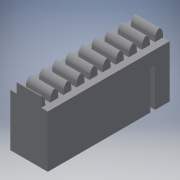
# Autodesk Inventor part: Alligator_Rack
Saved by Autodesk Inventor 2016 (Build 200138000, 138)
## iProperties
Created: 2017-05-22
Part Number: Alligator_Rack
Material: Generic
Document SubType Name: Modeling
Designer: nazardio000
Density: 1 g/cm^3
Appearance: Default
Author: nazardio000
Autodesk Inventor part; units mm, degrees
ref_plane "YZ Plane" through (0, 0, 0) normal (1, 0, 0) x (0, 1, 0)
ref_plane "XZ Plane" through (0, 0, 0) normal (0, 1, 0) x (-1, 0, 0)
ref_plane "XY Plane" through (0, 0, 0) normal (0, 0, 1) x (1, 0, 0)
sketch "Sketch2" plane through (0, 0, 0) normal (1, 0, 0) x (0, 1, 0)
  line L0 (-5.5245, 31.75) -> (-5.5245, -31.75)
  line L1 (-5.5245, -31.75) -> (5.5245, -31.75)
  line L2 (5.5245, -31.75) -> (5.5245, 31.75)
  line L3 (5.5245, 31.75) -> (-5.5245, 31.75)
  line L4 (-5.5245, 31.75) -> (5.5245, -31.75) construction
  line L5 (-5.5245, -31.75) -> (5.5245, 31.75) construction
  point P0 (0, 0)
  dimension "d4" = 63.5
  dimension "d5" = 11.049
  constraints: 12 end point, 2 midpoint, 2 parallel, 1 perpendicular, 1 vertical
  measures "d4" distance of L0.start L0.end
  measures "d5" distance of L1.end L0.end
extrude "Extrusion2" add sketch "Sketch2" along normal mid plane 9.779
sketch "Sketch3" plane through (0, 0, 0) normal (1, 0, 0) x (0, 1, 0)
  line L0 (5.5245, -31.75) -> (5.5245, 31.75) projected
  line L1 (5.5245, 31.9532) -> (5.5245, 29.4132)
  line L2 (5.5245, 31.9532) -> (5.5245, 29.4132)
  arc A0 (8.0645, 30.8543) -> (6.7945, 31.629) centre (6.3804, 29.5218) ccw
  line L3 (8.0645, 30.6737) -> (7.6408, 30.6737)
  arc A1 (6.7945, 29.7184) -> (8.0645, 30.4931) centre (6.3804, 31.8256) ccw
  line L4 (8.0645, 30.8543) -> (8.0645, 30.4931)
  line L5 (5.5245, 31.75) -> (5.5245, -31.75)
  arc A2 (8.0642, -1.6042) -> (8.0645, -1.6033) centre (6.6313, -1.0154) ccw
  line L6 (6.7945, 31.629) -> (5.5245, 31.7489)
  line L7 (6.7945, 29.7184) -> (5.5245, 29.5986)
  line L8 (5.5245, 31.7489) -> (6.7945, 31.629)
  line L9 (6.7945, 29.7184) -> (5.5245, 29.5986)
  line L10 (5.5245, 29.5986) -> (5.5245, 31.7489)
  arc A3 (8.0645, 30.8543) -> (6.7945, 31.629) centre (6.3804, 29.5218) ccw
  arc A4 (6.7945, 29.7184) -> (8.0645, 30.4931) centre (6.3804, 31.8256) ccw
  line L11 (8.0645, 30.8543) -> (8.0645, 30.4931)
  line L12 (8.0645, 27.2655) -> (7.6408, 27.2655)
  line L13 (8.0645, 27.4461) -> (8.0645, 27.0848)
  line L14 (8.0645, 27.4461) -> (8.0645, 27.0848)
  arc A5 (6.7945, 26.3101) -> (8.0645, 27.0848) centre (6.3804, 28.4173) ccw
  arc A6 (8.0645, 27.4461) -> (6.7945, 28.2208) centre (6.3804, 26.1136) ccw
  arc A7 (6.7945, 26.3101) -> (8.0645, 27.0848) centre (6.3804, 28.4173) ccw
  arc A8 (8.0645, 27.4461) -> (6.7945, 28.2208) centre (6.3804, 26.1136) ccw
  line L15 (5.5245, 28.3417) -> (5.5245, -35.1582)
  line L16 (5.5245, 28.5449) -> (5.5245, 26.0049)
  line L17 (6.7945, 26.3101) -> (5.5245, 26.1903)
  line L18 (5.5245, 28.3406) -> (6.7945, 28.2208)
  line L19 (6.7945, 26.3101) -> (5.5245, 26.1903)
  line L20 (5.5245, 26.1903) -> (5.5245, 28.3406)
  line L21 (5.5245, 28.5449) -> (5.5245, 26.0049)
  line L22 (6.7945, 28.2208) -> (5.5245, 28.3406)
  line L23 (8.0645, 23.8572) -> (7.6408, 23.8572)
  line L24 (8.0645, 24.0378) -> (8.0645, 23.6766)
  line L25 (8.0645, 24.0378) -> (8.0645, 23.6766)
  arc A9 (6.7945, 22.9019) -> (8.0645, 23.6766) centre (6.3804, 25.0091) ccw
  arc A10 (8.0645, 24.0378) -> (6.7945, 24.8125) centre (6.3804, 22.7053) ccw
  arc A11 (6.7945, 22.9019) -> (8.0645, 23.6766) centre (6.3804, 25.0091) ccw
  arc A12 (8.0645, 24.0378) -> (6.7945, 24.8125) centre (6.3804, 22.7053) ccw
  line L26 (5.5245, 24.9335) -> (5.5245, -38.5665)
  line L27 (5.5245, 25.1367) -> (5.5245, 22.5967)
  line L28 (6.7945, 22.9019) -> (5.5245, 22.782)
  line L29 (5.5245, 24.9324) -> (6.7945, 24.8125)
  line L30 (6.7945, 22.9019) -> (5.5245, 22.782)
  line L31 (5.5245, 22.782) -> (5.5245, 24.9324)
  line L32 (5.5245, 25.1367) -> (5.5245, 22.5967)
  line L33 (6.7945, 24.8125) -> (5.5245, 24.9324)
  line L34 (8.0645, 20.449) -> (7.6408, 20.449)
  line L35 (8.0645, 20.6296) -> (8.0645, 20.2683)
  line L36 (8.0645, 20.6296) -> (8.0645, 20.2683)
  arc A13 (6.7945, 19.4936) -> (8.0645, 20.2683) centre (6.3804, 21.6008) ccw
  arc A14 (8.0645, 20.6296) -> (6.7945, 21.4043) centre (6.3804, 19.2971) ccw
  arc A15 (6.7945, 19.4936) -> (8.0645, 20.2683) centre (6.3804, 21.6008) ccw
  arc A16 (8.0645, 20.6296) -> (6.7945, 21.4043) centre (6.3804, 19.2971) ccw
  line L37 (5.5245, 21.5252) -> (5.5245, -41.9747)
  line L38 (5.5245, 21.7284) -> (5.5245, 19.1884)
  line L39 (6.7945, 19.4936) -> (5.5245, 19.3738)
  line L40 (5.5245, 21.5241) -> (6.7945, 21.4043)
  line L41 (6.7945, 19.4936) -> (5.5245, 19.3738)
  line L42 (5.5245, 19.3738) -> (5.5245, 21.5241)
  line L43 (5.5245, 21.7284) -> (5.5245, 19.1884)
  line L44 (6.7945, 21.4043) -> (5.5245, 21.5241)
  line L45 (8.0645, 17.0407) -> (7.6408, 17.0407)
  line L46 (8.0645, 17.2213) -> (8.0645, 16.8601)
  line L47 (8.0645, 17.2213) -> (8.0645, 16.8601)
  arc A17 (6.7945, 16.0854) -> (8.0645, 16.8601) centre (6.3804, 18.1926) ccw
  arc A18 (8.0645, 17.2213) -> (6.7945, 17.996) centre (6.3804, 15.8888) ccw
  arc A19 (6.7945, 16.0854) -> (8.0645, 16.8601) centre (6.3804, 18.1926) ccw
  arc A20 (8.0645, 17.2213) -> (6.7945, 17.996) centre (6.3804, 15.8888) ccw
  line L48 (5.5245, 18.117) -> (5.5245, -45.383)
  line L49 (5.5245, 18.3202) -> (5.5245, 15.7802)
  line L50 (6.7945, 16.0854) -> (5.5245, 15.9655)
  line L51 (5.5245, 18.1159) -> (6.7945, 17.996)
  line L52 (6.7945, 16.0854) -> (5.5245, 15.9655)
  line L53 (5.5245, 15.9655) -> (5.5245, 18.1159)
  line L54 (5.5245, 18.3202) -> (5.5245, 15.7802)
  line L55 (6.7945, 17.996) -> (5.5245, 18.1159)
  line L56 (8.0645, 13.6324) -> (7.6408, 13.6324)
  line L57 (8.0645, 13.8131) -> (8.0645, 13.4518)
  line L58 (8.0645, 13.8131) -> (8.0645, 13.4518)
  arc A21 (6.7945, 12.6771) -> (8.0645, 13.4518) centre (6.3804, 14.7843) ccw
  arc A22 (8.0645, 13.8131) -> (6.7945, 14.5878) centre (6.3804, 12.4806) ccw
  arc A23 (6.7945, 12.6771) -> (8.0645, 13.4518) centre (6.3804, 14.7843) ccw
  arc A24 (8.0645, 13.8131) -> (6.7945, 14.5878) centre (6.3804, 12.4806) ccw
  line L59 (5.5245, 14.7087) -> (5.5245, -48.7912)
  line L60 (5.5245, 14.9119) -> (5.5245, 12.3719)
  line L61 (6.7945, 12.6771) -> (5.5245, 12.5573)
  line L62 (5.5245, 14.7076) -> (6.7945, 14.5878)
  line L63 (6.7945, 12.6771) -> (5.5245, 12.5573)
  line L64 (5.5245, 12.5573) -> (5.5245, 14.7076)
  line L65 (5.5245, 14.9119) -> (5.5245, 12.3719)
  line L66 (6.7945, 14.5878) -> (5.5245, 14.7076)
  line L67 (8.0645, 10.2242) -> (7.6408, 10.2242)
  line L68 (8.0645, 10.4048) -> (8.0645, 10.0436)
  line L69 (8.0645, 10.4048) -> (8.0645, 10.0436)
  arc A25 (6.7945, 9.2689) -> (8.0645, 10.0436) centre (6.3804, 11.3761) ccw
  arc A26 (8.0645, 10.4048) -> (6.7945, 11.1795) centre (6.3804, 9.0723) ccw
  arc A27 (6.7945, 9.2689) -> (8.0645, 10.0436) centre (6.3804, 11.3761) ccw
  arc A28 (8.0645, 10.4048) -> (6.7945, 11.1795) centre (6.3804, 9.0723) ccw
  line L70 (5.5245, 11.3005) -> (5.5245, -52.1995)
  line L71 (5.5245, 11.5037) -> (5.5245, 8.9637)
  line L72 (6.7945, 9.2689) -> (5.5245, 9.149)
  line L73 (5.5245, 11.2994) -> (6.7945, 11.1795)
  line L74 (6.7945, 9.2689) -> (5.5245, 9.149)
  line L75 (5.5245, 9.149) -> (5.5245, 11.2994)
  line L76 (5.5245, 11.5037) -> (5.5245, 8.9637)
  line L77 (6.7945, 11.1795) -> (5.5245, 11.2994)
  line L78 (8.0645, 6.8159) -> (7.6408, 6.8159)
  line L79 (8.0645, 6.9966) -> (8.0645, 6.6353)
  line L80 (8.0645, 6.9966) -> (8.0645, 6.6353)
  arc A29 (6.7945, 5.8606) -> (8.0645, 6.6353) centre (6.3804, 7.9678) ccw
  arc A30 (8.0645, 6.9966) -> (6.7945, 7.7713) centre (6.3804, 5.6641) ccw
  arc A31 (6.7945, 5.8606) -> (8.0645, 6.6353) centre (6.3804, 7.9678) ccw
  arc A32 (8.0645, 6.9966) -> (6.7945, 7.7713) centre (6.3804, 5.6641) ccw
  line L81 (5.5245, 7.8922) -> (5.5245, -55.6077)
  line L82 (5.5245, 8.0954) -> (5.5245, 5.5554)
  line L83 (6.7945, 5.8606) -> (5.5245, 5.7408)
  line L84 (5.5245, 7.8911) -> (6.7945, 7.7713)
  line L85 (6.7945, 5.8606) -> (5.5245, 5.7408)
  line L86 (5.5245, 5.7408) -> (5.5245, 7.8911)
  line L87 (5.5245, 8.0954) -> (5.5245, 5.5554)
  line L88 (6.7945, 7.7713) -> (5.5245, 7.8911)
  line L89 (8.0645, 3.4077) -> (7.6408, 3.4077)
  line L90 (8.0645, 3.5883) -> (8.0645, 3.2271)
  line L91 (8.0645, 3.5883) -> (8.0645, 3.2271)
  arc A33 (6.7945, 2.4524) -> (8.0645, 3.2271) centre (6.3804, 4.5596) ccw
  arc A34 (8.0645, 3.5883) -> (6.7945, 4.363) centre (6.3804, 2.2558) ccw
  arc A35 (6.7945, 2.4524) -> (8.0645, 3.2271) centre (6.3804, 4.5596) ccw
  arc A36 (8.0645, 3.5883) -> (6.7945, 4.363) centre (6.3804, 2.2558) ccw
  line L92 (5.5245, 4.484) -> (5.5245, -59.016)
  line L93 (5.5245, 4.6872) -> (5.5245, 2.1472)
  line L94 (6.7945, 2.4524) -> (5.5245, 2.3325)
  line L95 (5.5245, 4.4829) -> (6.7945, 4.363)
  line L96 (6.7945, 2.4524) -> (5.5245, 2.3325)
  line L97 (5.5245, 2.3325) -> (5.5245, 4.4829)
  line L98 (5.5245, 4.6872) -> (5.5245, 2.1472)
  line L99 (6.7945, 4.363) -> (5.5245, 4.4829)
  line L100 (8.0645, -0.0006) -> (7.6408, -0.0006)
  line L101 (8.0645, 0.1801) -> (8.0645, -0.1812)
  line L102 (8.0645, 0.1801) -> (8.0645, -0.1812)
  arc A37 (6.7945, -0.9559) -> (8.0645, -0.1812) centre (6.3804, 1.1513) ccw
  arc A38 (8.0645, 0.1801) -> (6.7945, 0.9548) centre (6.3804, -1.1524) ccw
  arc A39 (6.7945, -0.9559) -> (8.0645, -0.1812) centre (6.3804, 1.1513) ccw
  arc A40 (8.0645, 0.1801) -> (6.7945, 0.9548) centre (6.3804, -1.1524) ccw
  line L103 (5.5245, 1.0757) -> (5.5245, -62.4242)
  line L104 (5.5245, 1.2789) -> (5.5245, -1.2611)
  line L105 (6.7945, -0.9559) -> (5.5245, -1.0757)
  line L106 (5.5245, 1.0746) -> (6.7945, 0.9548)
  line L107 (6.7945, -0.9559) -> (5.5245, -1.0757)
  line L108 (5.5245, -1.0757) -> (5.5245, 1.0746)
  line L109 (5.5245, 1.2789) -> (5.5245, -1.2611)
  line L110 (6.7945, 0.9548) -> (5.5245, 1.0746)
  line L111 (8.0645, -3.4088) -> (7.6408, -3.4088)
  line L112 (8.0645, -3.2282) -> (8.0645, -3.5894)
  line L113 (8.0645, -3.2282) -> (8.0645, -3.5894)
  arc A41 (6.7945, -4.3641) -> (8.0645, -3.5894) centre (6.3804, -2.2569) ccw
  arc A42 (8.0645, -3.2282) -> (6.7945, -2.4535) centre (6.3804, -4.5607) ccw
  arc A43 (6.7945, -4.3641) -> (8.0645, -3.5894) centre (6.3804, -2.2569) ccw
  arc A44 (8.0645, -3.2282) -> (6.7945, -2.4535) centre (6.3804, -4.5607) ccw
  line L114 (5.5245, -2.3325) -> (5.5245, -65.8325)
  line L115 (5.5245, -2.1293) -> (5.5245, -4.6693)
  line L116 (6.7945, -4.3641) -> (5.5245, -4.484)
  line L117 (5.5245, -2.3337) -> (6.7945, -2.4535)
  line L118 (6.7945, -4.3641) -> (5.5245, -4.484)
  line L119 (5.5245, -4.484) -> (5.5245, -2.3337)
  line L120 (5.5245, -2.1293) -> (5.5245, -4.6693)
  line L121 (6.7945, -2.4535) -> (5.5245, -2.3337)
  line L122 (8.0645, -6.8171) -> (7.6408, -6.8171)
  line L123 (8.0645, -6.6364) -> (8.0645, -6.9977)
  line L124 (8.0645, -6.6364) -> (8.0645, -6.9977)
  arc A45 (6.7945, -7.7724) -> (8.0645, -6.9977) centre (6.3804, -5.6652) ccw
  arc A46 (8.0645, -6.6364) -> (6.7945, -5.8617) centre (6.3804, -7.9689) ccw
  arc A47 (6.7945, -7.7724) -> (8.0645, -6.9977) centre (6.3804, -5.6652) ccw
  arc A48 (8.0645, -6.6364) -> (6.7945, -5.8617) centre (6.3804, -7.9689) ccw
  line L125 (5.5245, -5.7408) -> (5.5245, -69.2407)
  line L126 (5.5245, -5.5376) -> (5.5245, -8.0776)
  line L127 (6.7945, -7.7724) -> (5.5245, -7.8922)
  line L128 (5.5245, -5.7419) -> (6.7945, -5.8617)
  line L129 (6.7945, -7.7724) -> (5.5245, -7.8922)
  line L130 (5.5245, -7.8922) -> (5.5245, -5.7419)
  line L131 (5.5245, -5.5376) -> (5.5245, -8.0776)
  line L132 (6.7945, -5.8617) -> (5.5245, -5.7419)
  line L133 (8.0645, -10.2253) -> (7.6408, -10.2253)
  line L134 (8.0645, -10.0447) -> (8.0645, -10.4059)
  line L135 (8.0645, -10.0447) -> (8.0645, -10.4059)
  arc A49 (6.7945, -11.1806) -> (8.0645, -10.4059) centre (6.3804, -9.0734) ccw
  arc A50 (8.0645, -10.0447) -> (6.7945, -9.27) centre (6.3804, -11.3772) ccw
  arc A51 (6.7945, -11.1806) -> (8.0645, -10.4059) centre (6.3804, -9.0734) ccw
  arc A52 (8.0645, -10.0447) -> (6.7945, -9.27) centre (6.3804, -11.3772) ccw
  line L136 (5.5245, -9.149) -> (5.5245, -72.649)
  line L137 (5.5245, -8.9458) -> (5.5245, -11.4858)
  line L138 (6.7945, -11.1806) -> (5.5245, -11.3005)
  line L139 (5.5245, -9.1502) -> (6.7945, -9.27)
  line L140 (6.7945, -11.1806) -> (5.5245, -11.3005)
  line L141 (5.5245, -11.3005) -> (5.5245, -9.1502)
  line L142 (5.5245, -8.9458) -> (5.5245, -11.4858)
  line L143 (6.7945, -9.27) -> (5.5245, -9.1502)
  line L144 (8.0645, -13.6336) -> (7.6408, -13.6336)
  line L145 (8.0645, -13.4529) -> (8.0645, -13.8142)
  line L146 (8.0645, -13.4529) -> (8.0645, -13.8142)
  arc A53 (6.7945, -14.5889) -> (8.0645, -13.8142) centre (6.3804, -12.4817) ccw
  arc A54 (8.0645, -13.4529) -> (6.7945, -12.6782) centre (6.3804, -14.7854) ccw
  arc A55 (6.7945, -14.5889) -> (8.0645, -13.8142) centre (6.3804, -12.4817) ccw
  arc A56 (8.0645, -13.4529) -> (6.7945, -12.6782) centre (6.3804, -14.7854) ccw
  line L147 (5.5245, -12.5573) -> (5.5245, -76.0572)
  line L148 (5.5245, -12.3541) -> (5.5245, -14.8941)
  line L149 (6.7945, -14.5889) -> (5.5245, -14.7087)
  line L150 (5.5245, -12.5584) -> (6.7945, -12.6782)
  line L151 (6.7945, -14.5889) -> (5.5245, -14.7087)
  line L152 (5.5245, -14.7087) -> (5.5245, -12.5584)
  line L153 (5.5245, -12.3541) -> (5.5245, -14.8941)
  line L154 (6.7945, -12.6782) -> (5.5245, -12.5584)
  line L155 (8.0645, -17.0418) -> (7.6408, -17.0418)
  line L156 (8.0645, -16.8612) -> (8.0645, -17.2224)
  line L157 (8.0645, -16.8612) -> (8.0645, -17.2224)
  arc A57 (6.7945, -17.9971) -> (8.0645, -17.2224) centre (6.3804, -15.8899) ccw
  arc A58 (8.0645, -16.8612) -> (6.7945, -16.0865) centre (6.3804, -18.1937) ccw
  arc A59 (6.7945, -17.9971) -> (8.0645, -17.2224) centre (6.3804, -15.8899) ccw
  arc A60 (8.0645, -16.8612) -> (6.7945, -16.0865) centre (6.3804, -18.1937) ccw
  line L158 (5.5245, -15.9655) -> (5.5245, -79.4655)
  line L159 (5.5245, -15.7623) -> (5.5245, -18.3023)
  line L160 (6.7945, -17.9971) -> (5.5245, -18.117)
  line L161 (5.5245, -15.9667) -> (6.7945, -16.0865)
  line L162 (6.7945, -17.9971) -> (5.5245, -18.117)
  line L163 (5.5245, -18.117) -> (5.5245, -15.9667)
  line L164 (5.5245, -15.7623) -> (5.5245, -18.3023)
  line L165 (6.7945, -16.0865) -> (5.5245, -15.9667)
  line L166 (8.0645, -20.4501) -> (7.6408, -20.4501)
  line L167 (8.0645, -20.2694) -> (8.0645, -20.6307)
  line L168 (8.0645, -20.2694) -> (8.0645, -20.6307)
  arc A61 (6.7945, -21.4054) -> (8.0645, -20.6307) centre (6.3804, -19.2982) ccw
  arc A62 (8.0645, -20.2694) -> (6.7945, -19.4947) centre (6.3804, -21.6019) ccw
  arc A63 (6.7945, -21.4054) -> (8.0645, -20.6307) centre (6.3804, -19.2982) ccw
  arc A64 (8.0645, -20.2694) -> (6.7945, -19.4947) centre (6.3804, -21.6019) ccw
  line L169 (5.5245, -19.3738) -> (5.5245, -82.8737)
  line L170 (5.5245, -19.1706) -> (5.5245, -21.7106)
  line L171 (6.7945, -21.4054) -> (5.5245, -21.5252)
  line L172 (5.5245, -19.3749) -> (6.7945, -19.4947)
  line L173 (6.7945, -21.4054) -> (5.5245, -21.5252)
  line L174 (5.5245, -21.5252) -> (5.5245, -19.3749)
  line L175 (5.5245, -19.1706) -> (5.5245, -21.7106)
  line L176 (6.7945, -19.4947) -> (5.5245, -19.3749)
  line L177 (8.0645, -23.8583) -> (7.6408, -23.8583)
  line L178 (8.0645, -23.6777) -> (8.0645, -24.0389)
  line L179 (8.0645, -23.6777) -> (8.0645, -24.0389)
  arc A65 (6.7945, -24.8136) -> (8.0645, -24.0389) centre (6.3804, -22.7064) ccw
  arc A66 (8.0645, -23.6777) -> (6.7945, -22.903) centre (6.3804, -25.0102) ccw
  arc A67 (6.7945, -24.8136) -> (8.0645, -24.0389) centre (6.3804, -22.7064) ccw
  arc A68 (8.0645, -23.6777) -> (6.7945, -22.903) centre (6.3804, -25.0102) ccw
  line L180 (5.5245, -22.782) -> (5.5245, -86.282)
  line L181 (5.5245, -22.5788) -> (5.5245, -25.1188)
  line L182 (6.7945, -24.8136) -> (5.5245, -24.9335)
  line L183 (5.5245, -22.7832) -> (6.7945, -22.903)
  line L184 (6.7945, -24.8136) -> (5.5245, -24.9335)
  line L185 (5.5245, -24.9335) -> (5.5245, -22.7832)
  line L186 (5.5245, -22.5788) -> (5.5245, -25.1188)
  line L187 (6.7945, -22.903) -> (5.5245, -22.7832)
  line L188 (8.0645, -27.2666) -> (7.6408, -27.2666)
  line L189 (8.0645, -27.0859) -> (8.0645, -27.4472)
  line L190 (8.0645, -27.0859) -> (8.0645, -27.4472)
  arc A69 (6.7945, -28.2219) -> (8.0645, -27.4472) centre (6.3804, -26.1147) ccw
  arc A70 (8.0645, -27.0859) -> (6.7945, -26.3112) centre (6.3804, -28.4184) ccw
  arc A71 (6.7945, -28.2219) -> (8.0645, -27.4472) centre (6.3804, -26.1147) ccw
  arc A72 (8.0645, -27.0859) -> (6.7945, -26.3112) centre (6.3804, -28.4184) ccw
  line L191 (5.5245, -26.1903) -> (5.5245, -89.6902)
  line L192 (5.5245, -25.9871) -> (5.5245, -28.5271)
  line L193 (6.7945, -28.2219) -> (5.5245, -28.3417)
  line L194 (5.5245, -26.1914) -> (6.7945, -26.3112)
  line L195 (6.7945, -28.2219) -> (5.5245, -28.3417)
  line L196 (5.5245, -28.3417) -> (5.5245, -26.1914)
  line L197 (5.5245, -25.9871) -> (5.5245, -28.5271)
  line L198 (6.7945, -26.3112) -> (5.5245, -26.1914)
  line L199 (8.0645, -30.6748) -> (7.6408, -30.6748)
  line L200 (8.0645, -30.4942) -> (8.0645, -30.8554)
  line L201 (8.0645, -30.4942) -> (8.0645, -30.8554)
  arc A73 (6.7945, -31.6301) -> (8.0645, -30.8554) centre (6.3804, -29.5229) ccw
  arc A74 (8.0645, -30.4942) -> (6.7945, -29.7195) centre (6.3804, -31.8267) ccw
  arc A75 (6.7945, -31.6301) -> (8.0645, -30.8554) centre (6.3804, -29.5229) ccw
  arc A76 (8.0645, -30.4942) -> (6.7945, -29.7195) centre (6.3804, -31.8267) ccw
  line L202 (5.5245, -29.5985) -> (5.5245, -93.0985)
  line L203 (5.5245, -29.3953) -> (5.5245, -31.9353)
  line L204 (6.7945, -31.6301) -> (5.5245, -31.75)
  line L205 (5.5245, -29.5997) -> (6.7945, -29.7195)
  line L206 (6.7945, -31.6301) -> (5.5245, -31.75)
  line L207 (5.5245, -31.75) -> (5.5245, -29.5997)
  line L208 (5.5245, -29.3953) -> (5.5245, -31.9353)
  line L209 (6.7945, -29.7195) -> (5.5245, -29.5997)
  point P0 (0, 0)
  point P1 (6.7953, 29.7185)
  point P2 (6.7953, 26.3103)
  point P3 (6.7953, 22.902)
  point P4 (6.7953, 19.4938)
  point P5 (6.7953, 16.0855)
  point P6 (6.7953, 12.6773)
  point P7 (6.7953, 9.269)
  point P8 (6.7953, 5.8608)
  point P9 (6.7953, 2.4525)
  point P10 (6.7953, -0.9557)
  point P11 (6.7953, -4.364)
  point P12 (6.7953, -7.7722)
  point P13 (6.7953, -11.1805)
  point P14 (6.7953, -14.5887)
  point P15 (6.7953, -17.997)
  point P16 (6.7953, -21.4052)
  point P17 (6.7953, -24.8135)
  point P18 (6.7953, -28.2217)
  point P19 (6.7953, -31.63)
  dimension "d9" = 2.3368
  dimension "d63" = 84.61
  dimension "d64" = 84.61
  dimension "d74" = 3.4082
  constraints: 382 end point, 173 point on circle, 77 centre point, 19 coincident, 5 collinear, 3 symmetric about line, 2 concentric, 2 vertical, 1 horizontal, 595 other
  measures "d9" distance of L0.end L1.end
  measures "d63" angle of L0 L6
  measures "d64" angle of L0 L7
  measures "d74" distance of L1.end L16.end
sketch "Sketch4" plane through (-4.8895, -5.5245, -31.75) normal (0, -1, 0) x (1, 0, 0)
  line L0 (2.032, 0.0016) -> (7.747, 0.0016) projected
  line L1 (4.8895, 0.0016) -> (6.7945, 0.0016)
  line L2 (4.8895, 0.0016) -> (2.9845, 0.0016)
  line L3 (6.7945, 0.0016) -> (2.032, 0.0016)
  line L4 (2.9845, -0.9507) -> (6.7945, -0.9507)
  line L5 (6.7945, -0.9507) -> (6.7945, 0.0016)
  line L6 (6.7945, 0.0016) -> (6.7945, 2.5416)
  line L7 (7.747, 2.5416) -> (2.032, 2.5416) projected
  line L8 (2.032, 2.5416) -> (0, 2.5416)
  line L9 (0, 63.5) -> (0, 0) projected
  line L10 (6.7945, 2.5416) -> (9.779, 2.5416)
  line L11 (9.779, 0) -> (9.779, 63.5) projected
  line L12 (9.779, 2.5416) -> (9.779, 3.8116)
  line L13 (9.779, 3.8116) -> (0, 3.8116)
  line L14 (0, 2.5416) -> (0, 3.8116)
  line L15 (2.9845, 0.0016) -> (2.9845, -0.9507)
  line L16 (2.9845, 0.0016) -> (2.9845, 2.5416)
  line L17 (2.032, 2.5416) -> (2.9845, 2.5416)
  point P0 (4.8895, 31.75)
  dimension "d28" = 1.905
  dimension "d29" = 1.905
  dimension "d31" = 2.54
  dimension "d32" = 1.27
  constraints: 28 end point, 9 point on line, 2 collinear, 2 perpendicular, 1 horizontal, 1 midpoint, 1 parallel, 1 vertical
  measures "d28" distance of L1.start L1.end
  measures "d29" distance of L1.start L2.end
  measures "d31" distance of L1.end L6.end
  measures "d32" distance of L10.end L12.end
extrude "Extrusion4" cut sketch "Sketch4" against normal blind 10.16
sketch "Sketch5" plane through (-4.8895, -5.5245, 31.75) normal (0, -1, 0) x (1, 0, 0)
  line L0 (0, -59.6884) -> (9.779, -59.6884) projected
  line L1 (9.779, 0) -> (9.779, -59.6884) projected
  line L2 (9.779, 0) -> (0, 0) projected
  line L3 (0, -59.6884) -> (0, 0) projected
  line L4 (2.9845, -60.9584) -> (0, -60.9584) projected
  line L5 (0, -63.5) -> (0, -60.9584) projected
  line L6 (0, -63.5) -> (2.9845, -63.5) projected
  line L7 (2.9845, -63.5) -> (2.9845, -60.9584) projected
  line L8 (9.779, -60.9584) -> (6.7945, -60.9584) projected
  line L9 (6.7945, -60.9584) -> (6.7945, -63.5) projected
  line L10 (6.7945, -63.5) -> (9.779, -63.5) projected
  line L11 (9.779, -60.9584) -> (9.779, -63.5) projected
  point P0 (4.8895, -31.75)
extrude "Extrusion6" add sketch "Sketch5" along normal blind 2.54
sketch "Sketch6" plane through (4.8895, 0, 0) normal (1, 0, 0) x (0, 0, -1)
  line L0 (31.75, 5.5245) -> (31.75, -8.0645) projected
  line L1 (27.9384, 4.6355) -> (31.75, 4.6355)
  line L2 (31.75, 4.6355) -> (31.75, 2.0955)
  line L3 (31.75, 2.0955) -> (27.9384, 2.0955)
  line L4 (27.9384, 2.0955) -> (27.9384, 4.6355)
  point P0 (0, 0)
  dimension "d60" = 2.54
  constraints: 8 end point, 2 parallel, 1 horizontal, 1 perpendicular, 1 point on line
  measures "d60" distance of L3.end L1.start
extrude "Extrusion7" add sketch "Sketch6" against normal blind 9.779
extrude "Extrusion8" add sketch "Sketch3" along normal mid plane 6.35 contours L0 L6 A0 L4 A1 L7 | L0 L18 A6 L13 A5 L17 | L0 L29 A10 L24 A9 L28 | L0 L40 A14 L35 A13 L39 | L0 L51 A18 L46 A17 L50 | L0 L62 A22 L57 A21 L61 | L0 L73 A26 L68 A25 L72 | L0 L84 A30 L79 A29 L83 | L0 L95 A34 L90 A33 L94 | L0 L117 A2 A42 L112 A41 L116 | L0 L128 A46 L123 A45 L127 | L0 L139 A50 L134 A49 L138 | L0 L150 A54 L145 A53 L149 | L0 L161 A58 L156 A57 L160 | L0 L172 A62 L167 A61 L171 | L0 L183 A66 L178 A65 L182 | L0 L194 A70 L189 A69 L193 | L0 L205 A74 L200 A73 L204 | L117 A42 A2 | A2 A37 L105 L0 | L0 L106 A38 L101 L100 A2 | L100 L101 A37 A2
sketch "Sketch7" plane through (4.8895, 0, 0) normal (1, 0, 0) x (0, 0, -1)
  line L0 (29.2084, 2.0955) -> (31.75, 2.0955) projected
  line L1 (27.9384, 2.0955) -> (27.9384, -8.0645) projected
  line L2 (29.2084, 2.0955) -> (27.9384, 2.0955)
  line L3 (27.9384, 2.0955) -> (27.9384, -8.0645)
  line L4 (27.9384, -8.0645) -> (29.2084, -8.0645)
  line L5 (29.2084, -8.0645) -> (29.2084, 2.0955)
  line L6 (27.9384, -8.0645) -> (26.6684, -8.0645)
  line L7 (26.6684, -8.0645) -> (26.6684, 2.0955)
  line L8 (26.6684, 2.0955) -> (27.9384, 2.0955)
  line L9 (27.9384, 2.0955) -> (27.9384, -8.0645)
  point P0 (0, 0)
  dimension "d81" = 1.27
  constraints: 16 end point, 4 parallel, 2 horizontal, 2 perpendicular
  measures "d81" distance of L7.end L8.end
extrude "Extrusion9" add sketch "Sketch7" against normal blind 9.779 contours L2 L5 L4 L1
sketch "Sketch8" plane through (4.8895, 0, 0) normal (1, 0, 0) x (0, 0, -1)
  line L0 (31.75, -8.0645) -> (29.2084, -8.0645) projected
  line L1 (31.75, -8.0645) -> (27.94, -8.0645)
  line L2 (-31.75, -8.0645) -> (31.75, -8.0645) projected
  line L3 (27.94, -8.0645) -> (26.67, -8.0645)
  line L4 (27.94, -8.0645) -> (27.94, 2.0955)
  line L5 (27.94, 2.0955) -> (26.67, 2.0955)
  line L6 (26.67, 2.0955) -> (26.67, -8.0645)
  point P0 (0, 0)
  dimension "d84" = 3.81
  dimension "d85" = 1.27
  dimension "d86" = 10.16
  constraints: 10 end point, 2 perpendicular, 2 point on line, 1 vertical
  measures "d84" distance of L0.start L1.end
  measures "d85" distance of L1.end L3.end
  measures "d86" distance of L1.end L4.end
extrude "Extrusion10" cut sketch "Sketch8" against normal blind 9.779
sketch "Sketch9" plane through (4.8895, -8.0645, -27.94) normal (0, 0, 1) x (1, 0, 0)
  line L0 (-6.7945, 0) -> (-6.7945, 10.16) projected
  line L1 (-2.9845, 10.16) -> (-6.7945, 10.16) projected
  line L2 (-2.9845, 10.16) -> (-2.9845, 0) projected
  line L3 (-2.9845, 0) -> (-6.7945, 0) projected
  point P0 (-4.8895, 8.0645)
extrude "Extrusion11" cut sketch "Sketch9" against normal blind 9.779
sketch "Sketch10" plane through (-4.8895, 0, 0) normal (-1, 0, 0) x (0, 0, 1)
  line L0 (0, 10.8635) -> (42.4338, 10.8635)
  line L1 (42.4338, 10.8635) -> (42.4338, -15.1476)
  line L2 (42.4338, -15.1476) -> (0, -15.1476)
  line L3 (0, -15.1476) -> (0, 10.8635)
  point P0 (0, 0)
  constraints: 8 end point, 2 parallel, 1 horizontal, 1 perpendicular
extrude "Extrusion12" cut sketch "Sketch10" against normal blind 25.4
body "Solid2"
